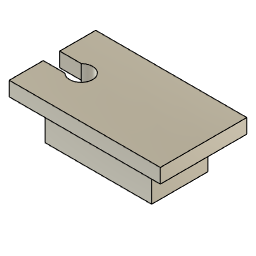
遮口 v2 (Autodesk Fusion 360 design; units mm, degrees)
Autodesk Fusion 360 part; units mm, degrees
sketch "草图1" plane through (0, 0, 0) normal (0, 0, 1) x (1, 0, 0)
  line L0 (0, 0) -> (14.8, 0)
  line L1 (14.8, 0) -> (14.8, 7.8)
  line L2 (14.8, 7.8) -> (0, 7.8)
  line L3 (0, 7.8) -> (0, 0)
  arc A0 (0, 2.7439) -> (0, 5.026) centre (1.1216, 3.885) ccw
  dimension "d1" = 14.8
  dimension "d2" = 7.8
  dimension "d3" = 3.2
  constraint horizontal L0
  constraint vertical L1
  constraint horizontal L2
  constraint vertical L3
  constraint coincident L0.start L3.end
  constraint coincident L3 A0.end
  constraint coincident L3 A0.start
  measures "d1" distance of L0.start L0.end
  measures "d2" distance of L0.start L2.end
  measures "d3" diameter of A0
extrude "拉伸1" add sketch "草图1" along normal blind 5 contours L0 L1 L2 L3 A0
sketch "草图2" plane through (0, 0, 5) normal (0, 0, 1) x (-1, 0, 0)
  line L0 (0, 0) -> (-14.8, 0)
  line L1 (-14.8, 0) -> (-14.8, -7.8)
  line L2 (-14.8, -7.8) -> (0, -7.8)
  line L3 (0, -7.8) -> (0, -5.026)
  arc A0 (0, -2.7439) -> (0, -5.026) centre (-1.1216, -3.885) ccw
  line L4 (0, -2.7439) -> (0, 0)
  line L5 (3, -10.0312) -> (-17.9802, -10.0312)
  line L6 (-17.9802, -10.0312) -> (-17.9802, 1.9802)
  line L7 (-17.9802, 1.9802) -> (3, 1.9802)
  line L8 (3, 1.9802) -> (3, -10.0312)
  constraint horizontal L5
  constraint vertical L6
  constraint horizontal L7
  constraint vertical L8
extrude "拉伸2" add sketch "草图2" along normal blind 2 contours L0 L1 L2 L3 A0 L4 | L5 L6 L7 L8
extrude "拉伸3" cut sketch "草图1" along normal blind 13 contours L3 A0
sketch "草图3" plane through (0, 0, 5) normal (0, 0, -1) x (1, 0, 0)
  line L0 (0, -5.026) -> (0, -2.7439)
  line L1 (0, -2.7439) -> (0, 0)
  line L2 (0, 0) -> (14.8, 0)
  line L3 (14.8, 0) -> (14.8, -7.8)
  line L4 (14.8, -7.8) -> (0, -7.8)
  line L5 (0, -7.8) -> (0, -5.026)
  line L6 (17.9802, 1.9802) -> (-3, 1.9802)
  line L7 (-3, 1.9802) -> (-3, -10.0312)
  line L8 (-3, -10.0312) -> (17.9802, -10.0312)
  line L9 (17.9802, -10.0312) -> (17.9802, 1.9802)
  line L10 (0, -2.7439) -> (-3, -2.7439)
  line L11 (0, -5.026) -> (-3, -5.026)
  constraint coincident L0.end L1.start
  constraint coincident L7 L10.end
  constraint perpendicular L7 L10
  constraint coincident L0.start L5.end
  constraint coincident L7 L11.end
  constraint perpendicular L7 L11
extrude "拉伸4" cut sketch "草图3" against normal blind 2 contours L0 L7 L10 L11
